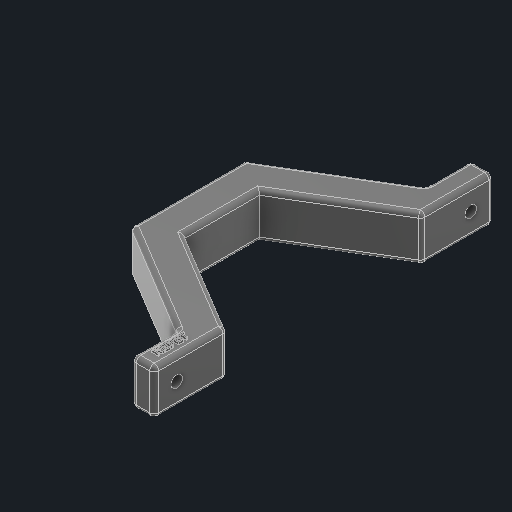
# Autodesk Inventor part: Soporte
Saved by Autodesk Inventor 2023 (Build 270158000, 158)
## iProperties
Created: 2023-11-13
Part Number: Soporte
Material: Acetal Resin, Black
Document SubType Name: Modeling
Designer: danie
Density: 1.425 g/cm^3
Appearance: Smooth - Black
Author: danie
Autodesk Inventor part; units mm, degrees
ref_plane "YZ Plane" through (0, 0, 0) normal (1, 0, 0) x (0, 1, 0)
ref_plane "XZ Plane" through (0, 0, 0) normal (0, 1, 0) x (-1, 0, 0)
ref_plane "XY Plane" through (0, 0, 0) normal (0, 0, 1) x (1, 0, 0)
sketch "Sketch1" plane through (0, 0, 0) normal (0, 1, 0) x (-1, 0, 0)
  line L0 (0, 0) -> (0, -150)
  line L1 (0, 0) -> (10, 0)
  line L2 (10, 0) -> (10, -20)
  line L3 (0, -75) -> (100, -75)
  line L4 (0, -150) -> (10, -150)
  line L5 (10, -150) -> (10, -130)
  line L6 (10, -20) -> (60, -50)
  line L7 (60, -50) -> (60, -75)
  line L8 (10, -130) -> (60, -100)
  line L9 (60, -100) -> (60, -75)
  line L10 (0, -31.4929) -> (45, -58.4929)
  line L11 (45, -58.4929) -> (45, -75)
  line L12 (0, -118.5071) -> (45, -91.5071)
  line L13 (45, -91.5071) -> (45, -75)
  point P0 (0, -118.5071)
  dimension "d0" = 150
  dimension "d1" = 10
  dimension "d2" = 20
  dimension "d3" = 100
  dimension "d27" = 25
  dimension "d28" = 15
  dimension "d29" = 15
  dimension "d31" = 50
  constraints: 28 end point, 5 symmetric about line, 3 perpendicular, 3 point on line, 2 horizontal, 1 midpoint, 1 parallel, 1 vertical
  measures "d0" distance of L0.start L0.end
  measures "d1" distance of L0.start L1.end
  measures "d2" distance of L1.end L2.end
  measures "d3" distance of L3.start L3.end
  measures "d27" distance of L6.end L7.end
  measures "d28" distance between parallel lines of L6 L10
  measures "d29" distance between parallel lines of L7 L11
  measures "d31" distance between parallel lines of L2 L7
extrude "Extrusion1" add sketch "Sketch1" along normal blind 20 contours L1 L2 L6 L7 L3 L11 L10 L0 | L12 L13 L3 L9 L8 L5 L4 L0
sketch "Sketch2" plane through (-10, 0, -20) normal (-1, 0, 0) x (0, 0, 1)
  line L0 (0, 0) -> (20, 0) projected
  line L1 (20, 0) -> (20, 20) projected
  line L2 (0, 20) -> (20, 20) projected
  line L3 (0, 0) -> (0, 20) projected
  line L4 (-130, 0) -> (-110, 0) projected
  line L5 (-110, 0) -> (-110, 20) projected
  line L6 (-130, 20) -> (-110, 20) projected
  line L7 (-130, 0) -> (-130, 20) projected
  line L8 (20, 0) -> (0, 0)
  line L9 (0, 0) -> (0, 20)
  line L10 (0, 20) -> (20, 20)
  line L11 (20, 20) -> (20, 0)
  line L12 (20, 20) -> (-130, 20) projected
  line L13 (-130, 20) -> (-110, 20)
  line L14 (-110, 20) -> (-110, 0)
  line L15 (-110, 0) -> (-130, 0)
  line L16 (-130, 0) -> (-130, 20)
  line L17 (20, 0) -> (-130, 0) projected
  line L18 (20, 0) -> (0, 20)
  line L19 (0, 0) -> (20, 20)
  line L20 (20, 20) -> (-130, 20) projected
  line L21 (-130, 20) -> (-110, 0)
  line L22 (-110, 20) -> (-130, 0)
  circle A0 centre (10, 10) radius 2.5
  circle A1 centre (-120, 10) radius 2.5
  point P0 (-90.4908, 20)
  point P1 (-9.5092, 0)
  point P2 (-9.5092, 20)
  dimension "d9" = 5
  constraints: 24 end point, 5 perpendicular, 4 parallel, 2 centre point, 2 horizontal, 2 midpoint, 1 point on line
  measures "d9" diameter of A0
hole "Hole2" at (-10, 10, -10) at (-10, 10, -140) direction (1, 0, 0) diameter 5 depth 10 counterbore diameter 8.5 counterbore depth 2
sketch "Sketch4" plane through (0, 20, 0) normal (0, 1, 0) x (1, 0, 0)
  line L0 (-6.6525, 5.288) -> (-6.6525, 22.2372) construction
  line L1 (-6.6525, 22.2372) -> (-2.8292, 22.2372) construction
  line L2 (-2.8292, 22.2372) -> (-2.8292, 5.288) construction
  line L3 (-2.8292, 5.288) -> (-6.6525, 5.288) construction
  line L4 (-10, 20) -> (-10, 0) projected
  line L5 (-3.6025, 5.6041) -> (-6.6525, 5.6041)
  line L6 (-6.6525, 5.6041) -> (-6.6525, 6.2016)
  line L7 (-6.6525, 6.2016) -> (-4.6068, 7.4546)
  line L8 (-4.6068, 7.4546) -> (-6.6525, 7.4546)
  line L9 (-6.6525, 7.4546) -> (-6.6525, 8.0241)
  line L10 (-6.6525, 8.0241) -> (-3.6025, 8.0241)
  line L11 (-3.6025, 8.0241) -> (-3.6025, 7.4081)
  line L12 (-3.6025, 7.4081) -> (-5.6041, 6.1737)
  line L13 (-5.6041, 6.1737) -> (-3.6025, 6.1737)
  line L14 (-3.6025, 6.1737) -> (-3.6025, 5.6041)
  line L15 (-3.6025, 8.6774) -> (-6.6525, 8.6774)
  line L16 (-6.6525, 8.6774) -> (-6.6525, 10.9393)
  line L17 (-6.6525, 10.9393) -> (-6.1364, 10.9393)
  line L18 (-6.1364, 10.9393) -> (-6.1364, 9.2934)
  line L19 (-6.1364, 9.2934) -> (-5.46, 9.2934)
  line L20 (-5.46, 9.2934) -> (-5.46, 10.8254)
  line L21 (-5.46, 10.8254) -> (-4.9439, 10.8254)
  line L22 (-4.9439, 10.8254) -> (-4.9439, 9.2934)
  line L23 (-4.9439, 9.2934) -> (-4.1186, 9.2934)
  line L24 (-4.1186, 9.2934) -> (-4.1186, 10.9974)
  line L25 (-4.1186, 10.9974) -> (-3.6025, 10.9974)
  line L26 (-3.6025, 10.9974) -> (-3.6025, 8.6774)
  line L27 (-3.6025, 11.5205) -> (-6.6525, 11.5205)
  line L28 (-6.6525, 11.5205) -> (-6.6525, 12.5085)
  spline S0 degree 2 poles (-6.6525, 12.5085) (-6.6525, 13.071) (-6.606, 13.2407) knots 0 0 0 1 1 1
  spline S1 degree 2 poles (-6.606, 13.2407) (-6.5386, 13.5034) (-6.0783, 13.8568) (-5.7134, 13.8568) knots 0 0 0 1 2 2 2
  spline S2 degree 2 poles (-5.7134, 13.8568) (-5.4344, 13.8568) (-5.0508, 13.6522) (-4.8323, 13.3384) (-4.7974, 13.1757) knots 0 0 0 1 2 3 3 3
  spline S3 degree 2 poles (-4.7974, 13.1757) (-4.7533, 12.9571) (-4.7533, 12.5387) knots 0 0 0 1 1 1
  line L29 (-4.7533, 12.5387) -> (-4.7533, 12.1365)
  line L30 (-4.7533, 12.1365) -> (-3.6025, 12.1365)
  line L31 (-3.6025, 12.1365) -> (-3.6025, 11.5205)
  line L32 (-6.1364, 12.1365) -> (-5.2693, 12.1365)
  line L33 (-5.2693, 12.1365) -> (-5.2693, 12.4736)
  spline S4 degree 2 poles (-5.2693, 12.4736) (-5.2693, 12.8386) (-5.3646, 13.0827) (-5.5692, 13.2221) (-5.7041, 13.2221) knots 0 0 0 1 2 3 3 3
  spline S5 degree 2 poles (-5.7041, 13.2221) (-5.8714, 13.2221) (-6.0876, 13.0269) (-6.1155, 12.8758) knots 0 0 0 1 2 2 2
  spline S6 degree 2 poles (-6.1155, 12.8758) (-6.1364, 12.7665) (-6.1364, 12.4341) knots 0 0 0 1 1 1
  line L34 (-6.1364, 12.4341) -> (-6.1364, 12.1365)
  line L35 (-3.6025, 14.3636) -> (-6.6525, 14.3636)
  line L36 (-6.6525, 14.3636) -> (-6.6525, 16.6255)
  line L37 (-6.6525, 16.6255) -> (-6.1364, 16.6255)
  line L38 (-6.1364, 16.6255) -> (-6.1364, 14.9796)
  line L39 (-6.1364, 14.9796) -> (-5.46, 14.9796)
  line L40 (-5.46, 14.9796) -> (-5.46, 16.5116)
  line L41 (-5.46, 16.5116) -> (-4.9439, 16.5116)
  line L42 (-4.9439, 16.5116) -> (-4.9439, 14.9796)
  line L43 (-4.9439, 14.9796) -> (-4.1186, 14.9796)
  line L44 (-4.1186, 14.9796) -> (-4.1186, 16.6836)
  line L45 (-4.1186, 16.6836) -> (-3.6025, 16.6836)
  line L46 (-3.6025, 16.6836) -> (-3.6025, 14.3636)
  line L47 (-3.6025, 17.8925) -> (-6.1364, 17.8925)
  line L48 (-6.1364, 17.8925) -> (-6.1364, 16.9882)
  line L49 (-6.1364, 16.9882) -> (-6.6525, 16.9882)
  line L50 (-6.6525, 16.9882) -> (-6.6525, 19.4105)
  line L51 (-6.6525, 19.4105) -> (-6.1364, 19.4105)
  line L52 (-6.1364, 19.4105) -> (-6.1364, 18.5085)
  line L53 (-6.1364, 18.5085) -> (-3.6025, 18.5085)
  line L54 (-3.6025, 18.5085) -> (-3.6025, 17.8925)
  point P0 (0, 0)
  point P1 (-8, 18.7326)
  constraints: 1 parallel, 2 other
emboss "Emboss1" sketch "Sketch4" operation add depth 1 direction (0, -1, 0)
fillet "Fillet3" radius 2 33 edges at (-10, 10, -130) (-10, 10, -20) (-60, 20, -75) (-35, 20, -35) (-35, 20, -115) (-60, 10, -100) (-60, 10, -50) (-45, 20, -75) (-22.5, 20, -44.9929) (-22.5, 20, -105.0071) (-22.5, 0, -44.9929) (-35, 0, -35) (-22.5, 0, -105.0071) (-45, 0, -75) (-35, 0, -115) (-10, 0, -140) (0, 0, -134.2536) (0, 0, -15.7464) (-10, 0, -10) (-5, 0, 0) (-5, 0, -150) (-10, 10, 0) (-10, 10, -150) (-10, 20, -140) (-10, 20, -10) (-5, 20, 0) (0, 10, 0) (0, 20, -134.2536) (-5, 20, -150) (0, 10, -150) (0, 10, -118.5071) (0, 10, -31.4929) (0, 20, -15.7464)
body "Solid1"
